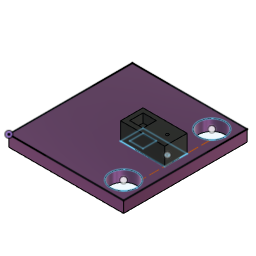
PAJ7620 (Autodesk Fusion 360 design; units mm, degrees)
Autodesk Fusion 360 part; units mm, degrees
sketch "Esquisse1" plane through (0, 0, 0) normal (0, 0, 1) x (1, 0, 0)
  line L0 (0, 0) -> (13, 0)
  line L1 (13, 0) -> (13, 14)
  line L2 (13, 14) -> (0, 14)
  line L3 (0, 14) -> (0, 0)
  circle A0 centre (11, 12) radius 1.5
  circle A1 centre (11, 2) radius 1.5
  line L4 (12, 8.2) -> (7, 8.2)
  line L5 (7, 8.2) -> (7, 5.66)
  line L6 (7, 5.66) -> (12, 5.66)
  line L7 (12, 5.66) -> (12, 8.2)
  line L8 (7.5, 7.7) -> (9, 7.7)
  line L9 (9, 7.7) -> (9, 6.2)
  line L10 (9, 6.2) -> (7.5, 6.2)
  line L11 (7.5, 6.2) -> (7.5, 7.7)
  circle A2 centre (11.0137, 6.95) radius 0.1606
  line L12 (11.9833, 10.8673) -> (11.9833, 3.1327) construction
  dimension "d1" = 13
  dimension "d2" = 14
  dimension "d3" = 3
  dimension "d4" = 3
  dimension "d5" = 5
  dimension "d6" = 2.54
  constraint horizontal L0
  constraint vertical L1
  constraint horizontal L2
  constraint vertical L3
  constraint coincident L0.start L3.end
  constraint horizontal L4
  constraint vertical L5
  constraint horizontal L6
  constraint vertical L7
  constraint horizontal L8
  constraint vertical L9
  constraint horizontal L10
  constraint vertical L11
  constraint coincident A0 L12.start
  constraint coincident A1 L12.end
  constraint perpendicular L6 L12
  measures "d1" distance of L0.start L0.end
  measures "d2" distance of L0.start L2.end
  measures "d3" diameter of A0
  measures "d4" diameter of A1
  measures "d5" distance of L4.start L4.end
  measures "d6" distance of L4.start L6.end
extrude "Extrusion1" add sketch "Esquisse1" against normal blind 1.27 contours L0 L1 L2 L3 | L4 L5 L6 L7 | L8 L9 L10 L11 makes body 1
extrude "Extrusion2" add sketch "Esquisse1" along normal blind 2 separate body contours L4 L5 L6 L7 makes body 2
extrude "Extrusion3" add sketch "Esquisse1" along normal blind 1 separate body contours L8 L9 L10 L11 makes body 3
